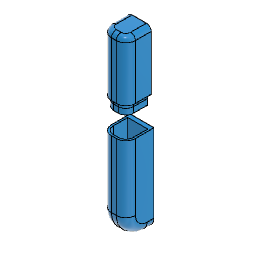
Tungsten Electrode Holder v1 (Autodesk Fusion 360 design; units mm, degrees)
Autodesk Fusion 360 part; units mm, degrees
sketch "Sketch1" plane through (0, 0, 0) normal (1, 0, 0) x (0, 1, 0)
  line L0 (20.0299, 48.5899) -> (-14.2601, 48.5899)
  line L1 (-14.2601, 48.5899) -> (-14.2601, -39.9829)
  line L2 (14.0071, -68.2501) -> (20.0299, -68.2501)
  line L3 (20.0299, -68.2501) -> (20.0299, 48.5899)
  line L4 (20.0299, 48.5899) -> (-12.8594, -31.1951) construction
  line L5 (-14.2601, 48.5899) -> (20.0299, -68.2501) construction
  arc A0 (-14.2601, -39.9829) -> (14.0071, -68.2501) centre (14.0071, -39.9829) ccw
  dimension "d42" = 116.84
  dimension "d43" = 34.29
  constraint horizontal L0
  constraint perpendicular L0 L1
  constraint parallel L0 L2
  constraint parallel L1 L3
  constraint coincident L4 origin
  constraint coincident L5 origin
  constraint tangent L1 A0
  constraint coincident A0 L4.end
  constraint tangent L2 A0
  measures "d42" distance of L0 L2
  measures "d43" distance of L1 L3
extrude "Extrude1" add sketch "Sketch1" along normal mid plane 31.75 makes body 1
fillet "Fillet1" radius 12.7 6 edges at (15.875, -14.2601, 4.3035) (15.875, -5.9808, -59.9708) (15.875, 17.0185, -68.2501) (-15.875, 17.0185, -68.2501) (-15.875, -5.9808, -59.9708) (-15.875, -14.2601, 4.3035) on bodies 1
shell "Shell1" thickness 2.54 removed faces 1 at (5.2917, 5.6366, 48.5899) on bodies 1
sketch "Sketch2" plane through (0, 20.0299, 0) normal (0, 1, 0) x (-1, 0, 0)
  arc A0 (3.175, -68.2501) -> (15.875, -55.5501) centre (3.175, -55.5501) ccw
  line L0 (15.875, -55.5501) -> (15.875, 48.5899)
  line L1 (15.875, 48.5899) -> (-15.875, 48.5899)
  line L2 (-15.875, 48.5899) -> (-15.875, -55.5501)
  arc A1 (-15.875, -55.5501) -> (-3.175, -68.2501) centre (-3.175, -55.5501) ccw
  line L3 (-3.175, -68.2501) -> (3.175, -68.2501)
  circle A2 centre (0, 27.8127) radius 3.0226
  circle A3 centre (0, -47.4729) radius 3.0226
  line L4 (0, 48.5899) -> (0, -68.2501) construction
  circle A4 centre (0, 2.7175) radius 3.0226
  circle A5 centre (0, -22.3777) radius 3.0226
  line L5 (0, -9.8301) -> (-15.875, -9.8301) construction
  line L6 (0, -22.3777) -> (0, 2.7175) construction
  point P0 (0, -9.8301)
  dimension "d11" = 6.0452
  dimension "d58" = 25.0952
  dimension "d60" = 25.0952
  dimension "d61" = 25.0952
  constraint equal A2 A3
  constraint midpoint L1 L4.start
  constraint midpoint L3 L4.end
  constraint coincident A3.centre L4
  constraint coincident A2.centre L4
  constraint coincident L4 A4.centre
  constraint equal A2 A4
  constraint coincident L4 A5.centre
  constraint equal A2 A5
  constraint midpoint L4 P0
  constraint coincident L2 L5.end
  constraint perpendicular L2 L5
  constraint coincident A5.centre L6.start
  constraint coincident A4.centre L6.end
  constraint midpoint L6 P0
  constraint coincident P0 L5.start
  measures "d11" diameter of A2
  measures "d58" distance of A4.centre A5.centre
  measures "d60" distance of A2.centre A4.centre
  measures "d61" distance of A3.centre A5.centre
extrude "Extrude2" add sketch "Sketch2" along normal blind 3.0861 bodies 1
copy_body "Body->Comp1" bodies 1 removing the originals makes body 2 in component "Tungsten Holder"
sketch "Sketch3" plane through (0, 0, 48.5899) normal (0, 0, 1) x (-1, 0, 0)
  line L0 (13.335, -17.4899) -> (-13.335, -17.4899)
  line L1 (-13.335, -17.4899) -> (-13.335, 1.5601)
  arc A0 (-3.175, 11.7201) -> (-13.335, 1.5601) centre (-3.175, 1.5601) ccw
  line L2 (-3.175, 11.7201) -> (3.175, 11.7201)
  arc A1 (13.335, 1.5601) -> (3.175, 11.7201) centre (3.175, 1.5601) ccw
  line L3 (13.335, 1.5601) -> (13.335, -17.4899)
  arc A2 (15.875, 1.5601) -> (3.175, 14.2601) centre (3.175, 1.5601) ccw
  line L4 (3.175, 14.2601) -> (-3.175, 14.2601)
  arc A3 (-3.175, 14.2601) -> (-15.875, 1.5601) centre (-3.175, 1.5601) ccw
  line L5 (-15.875, 1.5601) -> (-15.875, -23.116)
  line L6 (-15.875, -23.116) -> (15.875, -23.116)
  line L7 (15.875, -23.116) -> (15.875, 1.5601)
extrude "Extrude1'" add sketch "Sketch3" along normal blind 78.74 separate body contours L0 L1 A0 L2 A1 L3 | A2 L4 A3 L5 L6 L7 makes body 3 in component "Holder Cap"
fillet "Fillet1'" radius 6.35 5 edges at (-15.875, 10.778, 127.3299) (-12.1553, -10.5403, 127.3299) (0, -14.2601, 127.3299) (12.1553, -10.5403, 127.3299) (15.875, 10.778, 127.3299) on bodies 3 in component "Holder Cap"
extrude "Extrude2'" cut 1 faces at (5.2917, 23.116, 72.7199) along direction (0, -1, 0) blind 3.1242 on bodies 3 bodies 3 in component "Holder Cap"
sketch "Sketch4" plane through (-27.0606, 39.3147, 48.5899) normal (0, 0, -1) x (1, 0, 0)
  line L0 (11.1856, 19.3229) -> (42.9356, 19.3229)
  line L1 (42.9356, 19.3229) -> (42.9356, 40.8748)
  arc A0 (42.9356, 40.8748) -> (30.2356, 53.5748) centre (30.2356, 40.8748) ccw
  line L2 (30.2356, 53.5748) -> (23.8856, 53.5748)
  arc A1 (23.8856, 53.5748) -> (11.1856, 40.8748) centre (23.8856, 40.8748) ccw
  line L3 (11.1856, 40.8748) -> (11.1856, 19.3229)
  line L4 (13.7256, 21.8629) -> (40.3956, 21.8629)
  line L5 (40.3956, 21.8629) -> (40.3956, 40.8748)
  arc A2 (40.3956, 40.8748) -> (30.2356, 51.0348) centre (30.2356, 40.8748) ccw
  line L6 (30.2356, 51.0348) -> (23.8856, 51.0348)
  arc A3 (23.8856, 51.0348) -> (13.7256, 40.8748) centre (23.8856, 40.8748) ccw
  line L7 (13.7256, 40.8748) -> (13.7256, 21.8629)
  line L8 (14.9956, 23.1329) -> (39.1256, 23.1329)
  line L9 (39.1256, 23.1329) -> (39.1256, 40.8748)
  arc A4 (39.1256, 40.8748) -> (30.2356, 49.7648) centre (30.2356, 40.8748) ccw
  line L10 (30.2356, 49.7648) -> (23.8856, 49.7648)
  arc A5 (23.8856, 49.7648) -> (14.9956, 40.8748) centre (23.8856, 40.8748) ccw
  line L11 (14.9956, 40.8748) -> (14.9956, 23.1329)
  dimension "d23" = -2.54
  dimension "d24" = -3.81
shell "Shell1'" thickness 2.54 removed faces 1 at (-5.2917, 12.8079, 48.5899) on bodies 3 in component "Holder Cap"
sketch "Sketch6" plane through (0, 0, 48.5899) normal (0, 0, -1) x (1, 0, 0)
  line L0 (13.335, -17.4518) -> (-13.335, -17.4518)
  line L1 (-13.335, -17.4518) -> (-13.335, 1.5601)
  arc A0 (-3.175, 11.7201) -> (-13.335, 1.5601) centre (-3.175, 1.5601) ccw
  line L2 (-3.175, 11.7201) -> (3.175, 11.7201)
  arc A1 (13.335, 1.5601) -> (3.175, 11.7201) centre (3.175, 1.5601) ccw
  line L3 (13.335, 1.5601) -> (13.335, -17.4518)
  line L4 (-15.875, -19.9918) -> (15.875, -19.9918)
  line L5 (15.875, -19.9918) -> (15.875, 1.5601)
  arc A2 (15.875, 1.5601) -> (3.175, 14.2601) centre (3.175, 1.5601) ccw
  line L6 (3.175, 14.2601) -> (-3.175, 14.2601)
  arc A3 (-3.175, 14.2601) -> (-15.875, 1.5601) centre (-3.175, 1.5601) ccw
  line L7 (-15.875, 1.5601) -> (-15.875, -19.9918)
  line L8 (-11.811, -15.9278) -> (-11.811, 1.5601)
  arc A4 (-3.175, 10.1961) -> (-11.811, 1.5601) centre (-3.175, 1.5601) ccw
  line L9 (-3.175, 10.1961) -> (3.175, 10.1961)
  arc A5 (11.811, 1.5601) -> (3.175, 10.1961) centre (3.175, 1.5601) ccw
  line L10 (11.811, 1.5601) -> (11.811, -15.9278)
  line L11 (11.811, -15.9278) -> (-11.811, -15.9278)
  dimension "d31" = -1.524
extrude "Extrude4" add sketch "Sketch6" along normal blind 12.7 draft -1 separate body contours L0 L1 A0 L2 A1 L3 makes body 4
extrude "Extrude5" add 1 faces at (3.937, 16.9438, 48.5899) along direction (0, 0, 1) blind 3.81 on bodies 4 bodies 4
sketch "Sketch8" plane through (8.1653, 5.4246, 48.5899) normal (0, 0, -1) x (1, 0, 0)
  line L0 (5.1697, -12.0272) -> (-21.5003, -12.0272)
  line L1 (-21.5003, -12.0272) -> (-21.5003, 6.9847)
  arc A0 (-11.3403, 17.1447) -> (-21.5003, 6.9847) centre (-11.3403, 6.9847) ccw
  line L2 (-11.3403, 17.1447) -> (-4.9903, 17.1447)
  arc A1 (5.1697, 6.9847) -> (-4.9903, 17.1447) centre (-4.9903, 6.9847) ccw
  line L3 (5.1697, 6.9847) -> (5.1697, -12.0272)
  line L4 (-24.0403, -14.5672) -> (7.7097, -14.5672)
  line L5 (7.7097, -14.5672) -> (7.7097, 6.9847)
  arc A2 (7.7097, 6.9847) -> (-4.9903, 19.6847) centre (-4.9903, 6.9847) ccw
  line L6 (-4.9903, 19.6847) -> (-11.3403, 19.6847)
  arc A3 (-11.3403, 19.6847) -> (-24.0403, 6.9847) centre (-11.3403, 6.9847) ccw
  line L7 (-24.0403, 6.9847) -> (-24.0403, -14.5672)
  line L8 (-21.3479, -11.8748) -> (-21.3479, 6.9847)
  arc A4 (-11.3403, 16.9923) -> (-21.3479, 6.9847) centre (-11.3403, 6.9847) ccw
  line L9 (-11.3403, 16.9923) -> (-4.9903, 16.9923)
  arc A5 (5.0173, 6.9847) -> (-4.9903, 16.9923) centre (-4.9903, 6.9847) ccw
  line L10 (5.0173, 6.9847) -> (5.0173, -11.8748)
  line L11 (5.0173, -11.8748) -> (-21.3479, -11.8748)
  dimension "d46" = -0.1524
extrude "Extrude7" cut sketch "Sketch8" along normal blind 11.684 draft -0.75 contours L0 L1 A0 L2 A1 L3 bodies 4
combine "Combine2" operation add target body 3 tool bodies 4 in component "Holder Cap"
chamfer "Chamfer2" distance 1.524 angle 45 6 edges at (13.335, 7.9459, 52.3999) (10.3592, -8.7443, 52.3999) (0, -11.7201, 52.3999) (-10.3592, -8.7443, 52.3999) (-13.335, 7.9459, 52.3999) (0, 17.4518, 52.3999) on bodies 3 in component "Holder Cap"
chamfer "Chamfer3" distance 0.635 angle 45 5 edges at (15.875, 19.9918, 84.7849) (14.0151, 19.9918, 125.47) (0, 19.9918, 127.3299) (-14.0151, 19.9918, 125.47) (-15.875, 19.9918, 84.7849) on bodies 3 in component "Holder Cap"
sketch "Sketch7" plane through (0, 0, 48.5899) normal (0, 0, -1) x (1, 0, 0)
  line L0 (-15.875, -19.3568) -> (-15.24, -19.9918)
  line L1 (-15.24, -19.9918) -> (15.24, -19.9918)
  line L2 (15.24, -19.9918) -> (15.875, -19.3568)
  line L3 (15.875, -19.3568) -> (15.875, 1.5601)
  arc A0 (15.875, 1.5601) -> (3.175, 14.2601) centre (3.175, 1.5601) ccw
  line L4 (3.175, 14.2601) -> (-3.175, 14.2601)
  arc A1 (-3.175, 14.2601) -> (-15.875, 1.5601) centre (-3.175, 1.5601) ccw
  line L5 (-15.875, 1.5601) -> (-15.875, -19.3568)
  arc A2 (13.1826, 1.5601) -> (3.175, 11.5677) centre (3.175, 1.5601) ccw
  line L6 (13.1826, 1.5601) -> (13.1826, -17.2994)
  line L7 (13.1826, -17.2994) -> (-13.1826, -17.2994)
  line L8 (-13.1826, -17.2994) -> (-13.1826, 1.5601)
  arc A3 (-3.175, 11.5677) -> (-13.1826, 1.5601) centre (-3.175, 1.5601) ccw
  line L9 (-3.175, 11.5677) -> (3.175, 11.5677)
sketch "Sketch1 (2)" plane through (0, 23.116, 0) normal (0, 1, 0) x (-1, 0, 0) in component "Round Magnet"
  circle A0 centre (0, 27.8127) radius 3.0226
  circle A1 centre (0, 2.7175) radius 3.0226
  circle A2 centre (0, -47.4729) radius 3.0226
  line L0 (-3.175, -68.2501) -> (3.175, -68.2501)
  arc A3 (3.175, -68.2501) -> (15.875, -55.5501) centre (3.175, -55.5501) ccw
  line L1 (15.875, -55.5501) -> (15.875, 48.5899)
  line L2 (15.875, 48.5899) -> (-15.875, 48.5899)
  line L3 (-15.875, 48.5899) -> (-15.875, -55.5501)
  arc A4 (-15.875, -55.5501) -> (-3.175, -68.2501) centre (-3.175, -55.5501) ccw
  circle A5 centre (0, 2.7175) radius 3
  circle A6 centre (0, 27.8127) radius 3
  circle A7 centre (0, -47.4729) radius 3
  circle A8 centre (0, -22.3777) radius 3.0226
  circle A9 centre (0, -22.3777) radius 3
  dimension "d51" = 6
  constraint concentric A1 A5
  constraint concentric A0 A6
  constraint concentric A2 A7
  constraint equal A5 A6
  constraint equal A5 A7
  constraint concentric A8 A9
  constraint equal A5 A9
  measures "d51" diameter of A5
extrude "Extrude1''" add sketch "Sketch1 (2)" along normal blind -3.06 and the other way blind -0.05 separate body contours A5 | A6 | A7 | A9 makes body 5 at (-2.9963, 21.0927, -47.6225) makes body 6 at (-2.9963, 21.0927, 2.5679) makes body 7 at (-2.9963, 21.0927, 27.6631) makes body 8 at (-2.9963, 21.0927, -22.5273) in component "Component"
component "Holder Cap" placed x (1, 0, 0) y (0, 1, 0) z (0, 0, 1) at (0, 0, 40.288)
component "Tungsten Holder" placed x (1, 0, 0) y (0, 1, 0) z (0, 0, 1) at (0, 0, 0)
component "Magnets" placed x (1, 0, 0) y (0, 1, 0) z (0, 0, 1) at (0, 0, 0)
component "Round Magnet" placed x (1, 0, 0) y (0, 1, 0) z (0, 0, 1) at (0, 0, 0) in component "Magnets"
component "Component" placed x (1, 0, 0) y (0, 1, 0) z (0, 0, 1) at (0, 0, 0) in component "Round Magnet"
equation "height = 4.5 in"
equation "width = 1.25 in"
equation "hole = 1 in"
equation "d6 = width"
equation "d42 = height + 0.1 in"
equation "d43 = width + 0.1 in"
equation "d58 = 0.75 in + 0.238 in"
named bodies: "Tungston Holder", "Tungsten Holder", "Cap"
